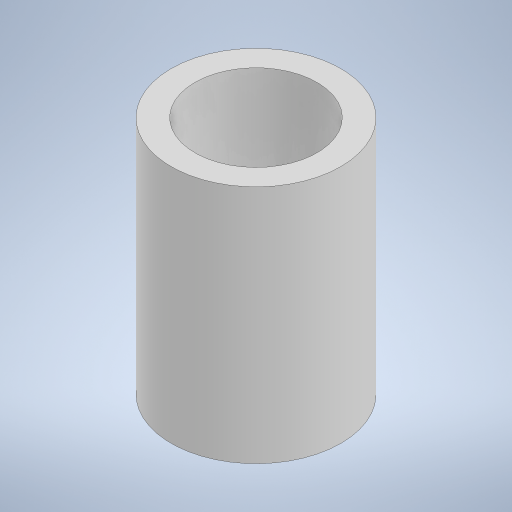
# Autodesk Inventor part: cell
Saved by Autodesk Inventor 2024.3 (Build 283343000, 343)
## iProperties
Created: 2025-09-23
Part Number: cell
Material: 일반
Document SubType Name: Modeling
Designer: joung
Density: 1 g/cm^3
Appearance: 기본값
Author: joung
Autodesk Inventor part; units mm, degrees
ref_plane "YZ Plane" through (0, 0, 0) normal (1, 0, 0) x (0, 1, 0)
ref_plane "XZ Plane" through (0, 0, 0) normal (0, 1, 0) x (-1, 0, 0)
ref_plane "XY Plane" through (0, 0, 0) normal (0, 0, 1) x (1, 0, 0)
sketch "스케치1" plane through (0, 0, 0) normal (0, 1, 0) x (-1, 0, 0)
  circle A0 centre (0, 0) radius 28.5
  circle A1 centre (0, 0) radius 20.5
  dimension "d0" = 57
  dimension "d1" = 8
  constraints: 2 centre point, 1 coincident
  measures "d0" diameter of A0
  measures "d1" radial gap between concentric circles of A0 A1
extrude "돌출1" add sketch "스케치1" along normal blind 80
sketch "스케치2" plane through (0, 0, 0) normal (0, -1, 0) x (1, 0, 0)
  circle A0 centre (0, 0) radius 28.5
  dimension "d6" = 57
  constraints: 1 centre point, 1 coincident
  measures "d6" diameter of A0
extrude "돌출2" add sketch "스케치2" along normal blind 0.5
